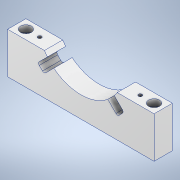
# Autodesk Inventor part: ODSY-0007-003
Saved by Autodesk Inventor 2021 (Build 250183000, 183)
## iProperties
Company: ERPL
Created: 2021-09-10
Material: Aluminum 6061
Document SubType Name: Modeling
Designer: ALEX CLAY
Density: 2.7 g/cm^3
Appearance: Aluminum - Flat
Mass: 599.899 g
Surface Area: 379.093 cm^2
Volume: 222.185 cm^3
Project: ODYSSEY
Description: ODYSSEY BOTTOM HOLDER
Part Number: ODSY-0007-003
Author: ALEX CLAY
Revision Number: 00
Autodesk Inventor part; units mm, degrees
ref_plane "YZ Plane" through (0, 0, 0) normal (1, 0, 0) x (0, 1, 0)
ref_plane "XZ Plane" through (0, 0, 0) normal (0, 1, 0) x (-1, 0, 0)
ref_plane "XY Plane" through (0, 0, 0) normal (0, 0, 1) x (1, 0, 0)
sketch "Sketch1" plane through (0, 0, 0) normal (0, 0, 1) x (1, 0, 0)
  arc A0 (-50.5454, 57.15) -> (50.5454, 57.15) centre (0, 88.9) ccw
  line L0 (-50.5454, 57.15) -> (-101.6, 57.15)
  line L1 (-101.6, 57.15) -> (-101.6, 0)
  line L2 (-101.6, 0) -> (101.6, 0)
  line L3 (101.6, 0) -> (101.6, 57.15)
  line L4 (101.6, 57.15) -> (50.5454, 57.15)
  line L5 (-142.24, 0) -> (142.24, 0) projected
  line L6 (0, 57.6383) -> (0, -27.9062) construction
  line L7 (0, -51.2675) -> (0, 112.2612) projected
  point P0 (0, 0)
  dimension "d32" = 57.15
  dimension "d33" = 59.69
  dimension "d63" = 88.9
  dimension "d64" = 203.2
  dimension "d65" = 101.6
  constraints: 12 end point, 4 perpendicular, 2 point on circle, 2 point on line, 1 centre point, 1 collinear, 1 horizontal, 1 midpoint, 1 vertical
  measures "d32" distance between parallel lines of L2 L4
  measures "d33" radius of A0
  measures "d63" distance from line of L5 A0.centre
  measures "d64" distance between parallel lines of L1 L3
  measures "d65" distance between parallel lines of L6 L1
extrude "Extrusion1" add sketch "Sketch1" along normal mid plane 25.4
sketch "Sketch2" plane through (-101.6, 57.15, 12.7) normal (0, 1, 0) x (1, 0, 0)
  line L0 (51.0546, 25.4) -> (51.0546, 0) projected
  line L1 (51.0546, 0) -> (0, 0) projected
  line L2 (152.1454, 25.4) -> (152.1454, 0) projected
  line L3 (203.2, 0) -> (152.1454, 0) projected
  line L4 (203.2, 25.4) -> (203.2, 0) projected
  line L5 (0, 0) -> (0, 25.4) projected
  point P0 (101.6, 12.7)
  point P1 (31.75, 12.7)
  point P2 (171.45, 12.7)
  dimension "d16" = 12.7
  dimension "d18" = 12.7
  dimension "d19" = 31.75
  dimension "d20" = 31.75
  measures "d16" distance from line of L1 point (31.75, 12.7)
  measures "d18" distance from line of L3 point (171.45, 12.7)
  measures "d19" distance from line of point (171.45, 12.7) L4
  measures "d20" distance from line of L5 point (31.75, 12.7)
hole "Hole1" at (-69.85, 57.15, 0) at (69.85, 57.15, 0) direction (0, -1, 0) diameter 4.9784 depth 25.4 thread size "1/4-20 UNC" class "2B" standard "ANSI Unified Screw Threads"
sketch "Sketch4" plane through (0, 0, 12.7) normal (0, 0, 1) x (1, 0, 0)
  line L0 (-46.4578, 51.4224) -> (-59.9282, 37.9521)
  line L1 (-59.9282, 37.9521) -> (-50.9479, 28.9718)
  line L2 (-50.9479, 28.9718) -> (-37.4776, 42.4422)
  line L3 (-37.4776, 42.4422) -> (-46.4578, 51.4224)
  line L4 (37.4776, 42.4422) -> (50.9479, 28.9718)
  line L5 (50.9479, 28.9718) -> (59.9282, 37.9521)
  line L6 (59.9282, 37.9521) -> (46.4578, 51.4224)
  line L7 (46.4578, 51.4224) -> (37.4776, 42.4422)
  line L8 (0, 53.9269) -> (0, 0) construction
  line L9 (-101.6, 0) -> (101.6, 0) projected
  arc A0 (-50.5454, 57.15) -> (50.5454, 57.15) centre (0, 88.9) ccw projected
  line L10 (34.6064, 54.2936) -> (52.2131, 36.6869) construction
  line L11 (-58.7882, 30.1118) -> (-24.955, 63.945) construction
  point P0 (46.4578, 51.4224)
  point P1 (-46.4578, 51.4224)
  dimension "d35" = 90
  dimension "d36" = 45
  dimension "d38" = 12.7
  dimension "d39" = 12.7
  dimension "d42" = 6.35
  dimension "d43" = 6.35
  dimension "d46" = 19.05
  dimension "d51" = 19.05
  constraints: 22 end point, 5 perpendicular, 2 point on circle, 2 point on line, 1 midpoint, 1 parallel, 1 vertical
  measures "d35" angle of L6 L0
  measures "d36" angle of L8 L0
  measures "d38" distance of L2.end L0.start
  measures "d39" distance of L6.end L4.start
  measures "d42" distance between parallel lines of L10 L4
  measures "d43" distance between parallel lines of L11 L0
  measures "d46" distance between parallel lines of L1 L3
  measures "d51" distance of L4.start L4.end
extrude "Extrusion2" cut sketch "Sketch4" against normal through all contours A0 L2 L1 L0 | A0 L6 L5 L4
sketch "Sketch3" plane through (50.5454, 57.15, 12.7) normal (0, 1, 0) x (1, 0, 0)
  line L0 (51.0546, 25.4) -> (51.0546, 0) projected
  line L1 (51.0546, 0) -> (0, 0) projected
  line L2 (-152.1454, 0) -> (-152.1454, 25.4) projected
  line L3 (-101.0907, 0) -> (-152.1454, 0) projected
  line L4 (-152.1454, 12.7) -> (51.0546, 12.7) construction
  point P0 (-50.5454, 12.7)
  point P1 (38.3546, 12.7)
  point P2 (-139.4454, 12.7)
  dimension "d28" = 12.7
  dimension "d30" = 12.7
  constraints: 2 end point, 2 midpoint, 2 point on line
  measures "d28" distance from line of point (38.355, 12.7) L0
  measures "d30" distance from line of L2 point (-139.445, 12.7)
hole "Hole2" at (88.9, 57.15, 0) at (-88.9, 57.15, 0) direction (0, -1, 0) diameter 8.89 end through all counterbore diameter 15.24 counterbore depth 8.89 clearance for "Socket Head Cap Screw" size "M8" standard "Ansi Metric M Profile"
fillet "Fillet2" radius 3.175 4 edges at (-59.9282, 37.9521, 0) (-50.9479, 28.9718, 0) (50.9479, 28.9718, 0) (59.9282, 37.9521, 0)
equation "\"d36\" = 0.5 * d35"
equation "\"d42\" = 0.5 * d39"
equation "\"d43\" = 0.5 * d38"
body "Solid1"
